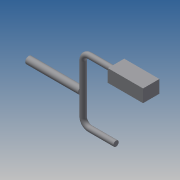
# Autodesk Inventor part: 槓桿
Saved by Autodesk Inventor 2015 (Build 190159000, 159)
## iProperties
Created: 2017-12-28
Part Number: 槓桿
Material: 一般
Document SubType Name: Modeling
Designer: user
Density: 1 g/cm^3
Appearance: 預設
Author: user
Autodesk Inventor part; units mm, degrees
ref_plane "YZ Plane" through (0, 0, 0) normal (1, 0, 0) x (0, 1, 0)
ref_plane "XZ Plane" through (0, 0, 0) normal (0, 1, 0) x (-1, 0, 0)
ref_plane "XY Plane" through (0, 0, 0) normal (0, 0, 1) x (1, 0, 0)
sketch "草圖1" plane through (0, 0, 0) normal (1, 0, 0) x (0, 1, 0)
  circle A0 centre (0, 0) radius 0.75
  dimension "d0" = 1.5
  constraints: 1 centre point, 1 coincident
  measures "d0" diameter of A0
sketch "草圖2" plane through (0, 0, 0) normal (0, 1, 0) x (-1, 0, 0)
  line L0 (0, 0) -> (7.3363, 0)
  line L1 (9.3363, -2) -> (9.3363, -8.9606)
  arc A0 (9.3363, -2) -> (7.3363, 0) centre (7.3363, -2) ccw
  point P0 (9.3363, 0)
  dimension "d3" = 2
  constraints: 4 end point, 2 point on circle, 2 point on line, 2 tangent, 1 centre point, 1 horizontal, 1 perpendicular
  measures "d3" radius of A0
sweep "掃掠1" add profiles "草圖1" path "草圖2" path curves L0 A0 L1
mirror "鏡射1" about plane through (-9.3363, 0, -8.9606) normal (0, 0, -1) of "掃掠1"
sketch "草圖3" plane through (0, 0, 0) normal (1, 0, 0) x (0, 1, 0)
  line L0 (-2.3279, -1.8091) -> (2.3279, -1.8091)
  line L1 (2.3279, -1.8091) -> (2.3279, 1.8091)
  line L2 (2.3279, 1.8091) -> (-2.3279, 1.8091)
  line L3 (-2.3279, 1.8091) -> (-2.3279, -1.8091)
  line L4 (-2.3279, -1.8091) -> (2.3279, 1.8091) construction
  line L5 (2.3279, -1.8091) -> (-2.3279, 1.8091) construction
  point P0 (0, 0)
  constraints: 12 end point, 2 midpoint, 2 parallel, 1 horizontal, 1 perpendicular
sketch "草圖4" plane through (0, 0, 0) normal (0, 1, 0) x (-1, 0, 0)
  line L0 (9.7833, -9.7316) -> (24.7833, -9.7316)
  line L1 (24.7833, -9.7316) -> (24.7833, -8.7316)
  line L2 (24.7833, -8.7316) -> (9.7833, -8.7316)
  line L3 (9.7833, -8.7316) -> (9.7833, -9.7316)
  point P0 (0, 0)
  point P1 (9.7833, -9.2316)
  dimension "d4" = 1
  dimension "d5" = 15
  constraints: 8 end point, 2 vertical, 1 horizontal, 1 midpoint, 1 parallel
  measures "d4" distance of L2.end L0.start
  measures "d5" distance of L1.end L2.end
revolve "迴轉1" add sketch "草圖4" angle 360 about axis through (-9.7833, 0, -9.7316) along (-1, 0, 0)
extrude "擠出1" add sketch "草圖3" along normal blind 10
